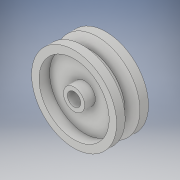
# Autodesk Inventor part: Rueda
Saved by Autodesk Inventor 2019 (Build 230136000, 136)
## iProperties
Created: 2019-05-14
Part Number: Rueda
Material: Generic
Document SubType Name: Modeling
Designer: Gustavo Marin
Density: 1 g/cm^3
Appearance: Default
Author: Gustavo Marin
Autodesk Inventor part; units mm, degrees
ref_plane "YZ Plane" through (0, 0, 0) normal (1, 0, 0) x (0, 1, 0)
ref_plane "XZ Plane" through (0, 0, 0) normal (0, 1, 0) x (-1, 0, 0)
ref_plane "XY Plane" through (0, 0, 0) normal (0, 0, 1) x (1, 0, 0)
sketch "Sketch1" plane through (0, 0, 0) normal (0, 1, 0) x (-1, 0, 0)
  line L0 (58.7375, 0) -> (58.7375, -38.1)
  line L1 (63.4971, -38.1) -> (63.5018, -25.4147)
  line L2 (63.5018, -25.4147) -> (92.7118, -25.4256)
  line L3 (92.7118, -25.4256) -> (92.7071, -38.1256)
  line L4 (92.7189, -0.0312) -> (92.7165, -12.7312)
  line L5 (92.7165, -12.7312) -> (63.5089, -12.7203)
  line L6 (63.5089, -12.7203) -> (63.5113, 0)
  line L7 (101.6, -10.1856) -> (92.7102, -19.0163)
  line L8 (92.7102, -19.0163) -> (101.6, -27.9656)
  line L9 (101.6, -38.1256) -> (92.7071, -38.1256)
  line L10 (63.4971, -38.1) -> (58.7375, -38.1)
  line L11 (58.7375, 0) -> (63.5113, 0)
  line L12 (92.7189, -0.0312) -> (101.6, -0.0312)
  line L13 (101.6, -0.0312) -> (101.6, -10.1856)
  line L14 (101.6, -27.9656) -> (101.6, -38.1256)
  line L15 (50.8042, 18.8171) -> (50.8042, -69.5336)
  point P0 (0, 0)
  point P1 (50.8042, -19.04)
  dimension "d8" = 41.91
  dimension "d9" = 12.7
  dimension "d15" = 90
  constraints: 32 end point, 6 parallel, 4 perpendicular, 2 horizontal, 2 point on line, 1 vertical
  measures "d8" distance from line of L3 point (50.804, -19.04)
  measures "d9" distance from line of L1 point (50.804, -19.04)
  measures "d15" angle of L7 L8
revolve "Revolution1" add sketch "Sketch1" angle 360 about axis through (-50.8042, 0, 18.8171) along (0, 0, -1)
body "Solid1"
